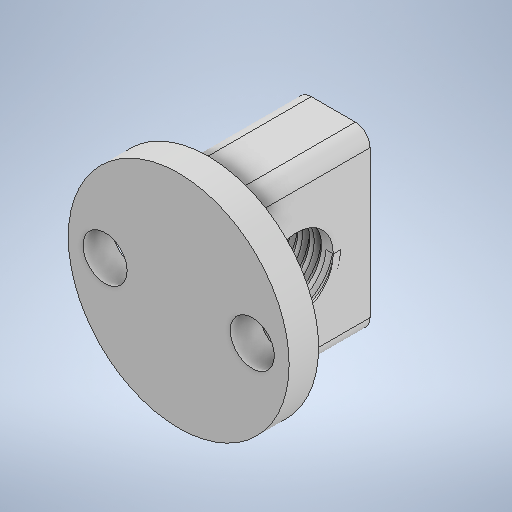
# Autodesk Inventor part: NUT
Saved by Autodesk Inventor 2025.2 (Build 292293000, 293)
## iProperties
Created: 2025-05-25
Part Number: NUT
Material: Generic
Document SubType Name: Modeling
Designer: Moaz
Density: 1 g/cm^3
Appearance: Default
Author: Moaz
Autodesk Inventor part; units mm, degrees
ref_plane "YZ Plane" through (0, 0, 0) normal (1, 0, 0) x (0, 1, 0)
ref_plane "XZ Plane" through (0, 0, 0) normal (0, 1, 0) x (-1, 0, 0)
ref_plane "XY Plane" through (0, 0, 0) normal (0, 0, 1) x (1, 0, 0)
sketch "Sketch1" plane through (0, 0, 0) normal (0, 0, 1) x (1, 0, 0)
  circle A0 centre (0, 0) radius 37.5
  circle A1 centre (-25, 0) radius 7.5
  circle A2 centre (25, 0) radius 7.5
  dimension "d0" = 75
  dimension "d1" = 15
  dimension "d2" = 15
  dimension "d3" = 25
  dimension "d4" = 25
  constraints: 3 centre point, 1 coincident
  measures "d0" diameter of A0
  measures "d1" diameter of A1
  measures "d2" diameter of A2
  measures "d3" distance of point (0, 0) A1.centre
  measures "d4" distance of point (0, 0) A2.centre
extrude "Extrusion1" add sketch "Sketch1" along normal blind 10
sketch "Sketch2" plane through (0, 0, 0) normal (0, 0, -1) x (-1, 0, 0)
  line L0 (7.5, -30) -> (-7.5, -30)
  line L1 (-12.5, -25) -> (-12.5, 25)
  line L2 (-7.5, 30) -> (7.5, 30)
  line L3 (12.5, 25) -> (12.5, -25)
  line L4 (12.5, -30) -> (-12.5, 30) construction
  line L5 (-12.5, -30) -> (12.5, 30) construction
  arc A0 (-7.5, 30) -> (-12.5, 25) centre (-7.5, 25) ccw
  arc A1 (-12.5, -25) -> (-7.5, -30) centre (-7.5, -25) ccw
  arc A2 (7.5, -30) -> (12.5, -25) centre (7.5, -25) ccw
  arc A3 (12.5, 25) -> (7.5, 30) centre (7.5, 25) ccw
  point P0 (0, 0)
  dimension "d10" = 25
  dimension "d11" = 60
  dimension "d12" = 5
  constraints: 12 end point, 8 point on circle, 8 point on line, 8 tangent, 4 centre point, 3 equal radius, 2 midpoint, 2 parallel, 1 horizontal, 1 perpendicular
  measures "d10" distance of L4.end L5.end
  measures "d11" distance of L5.start L4.end
  measures "d12" radius of A0
extrude "Extrusion2" add sketch "Sketch2" along normal blind 50
sketch "Sketch3" plane through (12.5, -25, 0) normal (1, 0, 0) x (0, 0, -1)
  circle A0 centre (25, 25) radius 12.5
  point P0 (0, 25)
  dimension "d15" = 25
  constraints: 1 centre point
  measures "d15" diameter of A0
extrude "Extrusion3" cut sketch "Sketch3" against normal blind 50
sketch "Sketch4" plane through (0, 0, 0) normal (0, 1, 0) x (-1, 0, 0)
  line L0 (-12.5, -37.5) -> (-12.5, -12.5) projected
  line L1 (-12.5, -37.5) -> (-10, -37.5)
  line L2 (-10, -37.5) -> (-10, -40)
  line L3 (-10, -40) -> (-12.5, -40)
  line L4 (-12.5, -40) -> (-12.5, -37.5)
  line L5 (-12.5, -25) -> (20.2126, -25)
  point P0 (0, 0)
  dimension "d18" = 2.5
  dimension "d19" = 2.5
  constraints: 10 end point, 2 horizontal, 2 parallel, 1 midpoint, 1 perpendicular
  measures "d18" distance of L2.end L3.end
  measures "d19" distance of L1.end L2.end
coil "Coil1" sketch "Sketch4" operation cut axis through (12.5, 0, -25) along (-1, 0, 0) pitch 4 turns 200 hand right
sketch "Sketch5" plane through (0, 0, 0) normal (0, 0, -1) x (-1, 0, 0)
  arc A0 (12.5, 25) -> (7.5, 30) centre (7.5, 25) ccw projected
  line L0 (12.5, 25) -> (12.5, -25) projected
  arc A1 (7.5, -30) -> (12.5, -25) centre (7.5, -25) ccw projected
  line L1 (7.5, -30) -> (-7.5, -30) projected
  arc A2 (-12.5, -25) -> (-7.5, -30) centre (-7.5, -25) ccw projected
  line L2 (-12.5, -25) -> (-12.5, 25) projected
  arc A3 (-7.5, 30) -> (-12.5, 25) centre (-7.5, 25) ccw projected
  line L3 (-7.5, 30) -> (7.5, 30) projected
  circle A4 centre (0, 0) radius 37.5 projected
  circle A5 centre (-25, 0) radius 7.5 projected
  circle A6 centre (25, 0) radius 7.5 projected
extrude "Extrusion4" add sketch "Sketch5" along normal blind 7.5
sketch "Sketch6" plane through (0, 0, 10) normal (0, 0, 1) x (1, 0, 0)
  circle A0 centre (0, 0) radius 37.5 projected
  circle A1 centre (25, 0) radius 7.5 projected
  circle A2 centre (-25, 0) radius 7.5 projected
extrude "Extrusion5" cut sketch "Sketch6" against normal blind 7.5
body "Solid1"
